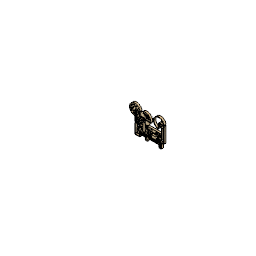
Peças - Texturitas Renders (Autodesk Fusion 360 design; units mm, degrees)
Autodesk Fusion 360 part; units mm, degrees
(part 1 of 2)
sketch "Sketch1" plane through (0, 0, 0) normal (0, 1, 0) x (1, 0, 0) in component "Peça P1"
  line L0 (36, 30) -> (-36, 30)
  line L1 (-40, 26) -> (-40, -6)
  line L2 (40, -6) -> (40, 26)
  arc A0 (-36, 30) -> (-40, 26) centre (-36, 26) ccw
  arc A1 (40, 26) -> (36, 30) centre (36, 26) ccw
  line L3 (-36, -10) -> (-25, -10)
  line L4 (25, -10) -> (36, -10)
  arc A2 (36, -10) -> (40, -6) centre (36, -6) ccw
  arc A3 (-40, -6) -> (-36, -10) centre (-36, -6) ccw
  line L5 (-35, 26) -> (-35, -6)
  line L6 (-38, -6) -> (-38, 26)
  arc A4 (-35, 26) -> (-38, 26) centre (-36.5, 26) ccw
  arc A5 (-38, -6) -> (-35, -6) centre (-36.5, -6) ccw
  line L7 (-30, 26) -> (-30, -6)
  line L8 (-33, -6) -> (-33, 26)
  arc A6 (-30, 26) -> (-33, 26) centre (-31.5, 26) ccw
  arc A7 (-33, -6) -> (-30, -6) centre (-31.5, -6) ccw
  line L9 (-20, 26) -> (-20, 12)
  line L10 (-23, 12) -> (-23, 26)
  arc A8 (-23, 12) -> (-20, 12) centre (-21.5, 12) ccw
  arc A9 (-20, 26) -> (-23, 26) centre (-21.5, 26) ccw
  line L11 (-15, 25) -> (-15, 15)
  line L12 (-18, 15) -> (-18, 25)
  arc A10 (-15, 25) -> (-18, 25) centre (-16.5, 25) ccw
  arc A11 (-18, 15) -> (-15, 15) centre (-16.5, 15) ccw
  line L13 (24.0859, 23.7871) -> (24.0859, 15.7871)
  line L14 (21.0859, 15.7871) -> (21.0859, 23.7871)
  arc A12 (24.0859, 23.7871) -> (21.0859, 23.7871) centre (22.5859, 23.7871) ccw
  arc A13 (21.0859, 15.7871) -> (24.0859, 15.7871) centre (22.5859, 15.7871) ccw
  line L15 (34, 25) -> (34, -5)
  line L16 (31, -5) -> (31, 25)
  arc A14 (34, 25) -> (31, 25) centre (32.5, 25) ccw
  arc A15 (31, -5) -> (34, -5) centre (32.5, -5) ccw
  line L17 (-21, -6) -> (-21, 6)
  arc A16 (-16, 11) -> (-21, 6) centre (-16, 6) ccw
  line L18 (-16, 11) -> (16, 11)
  arc A17 (21, 6) -> (16, 11) centre (16, 6) ccw
  line L19 (21, 6) -> (21, -6)
  arc A18 (-25, -10) -> (-21, -6) centre (-25, -6) ccw
  arc A19 (21, -6) -> (25, -10) centre (25, -6) ccw
  point P0 (-40, 30)
  point P1 (-40, -10)
  point P2 (40, -10)
  point P3 (-20, -10)
  point P4 (-20, 10)
  point P5 (20, 10)
  dimension "d1" = 80
  dimension "d2" = 40
  dimension "d3" = 40
  dimension "d4" = 20
  dimension "d5" = 4
  dimension "d6" = 4
  dimension "d9" = 4
  dimension "d10" = 4
  dimension "d79" = 1.5
  dimension "d80" = 16
  dimension "d81" = 52.5
  dimension "d82" = 47.5
  dimension "d83" = 37.5
  dimension "d84" = 32.5
  dimension "d85" = 16.5
  dimension "d86" = 11
  dimension "d87" = 9.7871
  dimension "d88" = 9
  dimension "d89" = 6.5859
  dimension "d91" = 3
  dimension "d92" = 30
  dimension "d93" = 8
  dimension "d166" = 4
  dimension "d167" = 4
  dimension "d375" = 6
  dimension "d376" = 12
  dimension "d377" = 6
  dimension "d378" = 5
  constraint horizontal L0
  constraint perpendicular L0 L1
  constraint parallel L0 L3
  constraint parallel L1 L2
  constraint coincident P0 L0
  constraint coincident P0 L1
  constraint tangent L0 A0
  constraint tangent L1 A0
  constraint tangent L0 A1
  constraint tangent L2 A1
  constraint collinear L3 L4
  constraint coincident P3 L3
  constraint coincident P2 L2
  constraint coincident P2 L4
  constraint tangent L2 A2
  constraint tangent L4 A2
  constraint coincident P1 L1
  constraint coincident P1 L3
  constraint tangent L1 A3
  constraint tangent L3 A3
  constraint vertical L5
  constraint vertical L6
  constraint tangent L6 A4
  constraint tangent L5 A5
  constraint vertical L7
  constraint vertical L8
  constraint tangent L8 A6
  constraint tangent L7 A7
  constraint vertical L9
  constraint vertical L10
  constraint tangent L10 A8
  constraint tangent L9 A9
  constraint vertical L11
  constraint vertical L12
  constraint tangent L11 A10
  constraint tangent L12 A11
  constraint vertical L13
  constraint vertical L14
  constraint tangent L13 A12
  constraint tangent L13 A13
  constraint vertical L15
  constraint vertical L16
  constraint tangent L15 A14
  constraint tangent L15 A15
  constraint tangent L6 A5
  constraint tangent L5 A4
  constraint tangent L8 A7
  constraint tangent L7 A6
  constraint tangent L10 A9
  constraint tangent L9 A8
  constraint tangent L12 A10
  constraint tangent L11 A11
  constraint tangent L14 A13
  constraint tangent L14 A12
  constraint tangent L16 A15
  constraint tangent L16 A14
  constraint collinear origin P3 P5
  constraint horizontal L1.end L6.start
  constraint horizontal L2.end L5.start
  constraint horizontal L1.end L8.start
  constraint horizontal L2.end L7.start
  constraint horizontal L2.end L9.start
  constraint horizontal L11.start L15.start
  constraint equal A4 A6
  constraint equal A4 A10
  constraint equal A4 A14
  constraint tangent A17 L19
  constraint tangent A16 L18
  constraint tangent L18 A17
  constraint tangent L17 A16
  constraint tangent L17 A18
  constraint tangent L3 A18
  constraint tangent L19 A19
  constraint tangent L4 A19
  constraint parallel L2 L17
  constraint parallel L0 L18
  constraint parallel L1 L19
  constraint equal A4 A8
  constraint equal A16 A17
  constraint equal L3 L4
  constraint equal L1 L18
  constraint vertical P3 L9.end
  constraint vertical P3 P4
  measures "d1" distance of P1 P2
  measures "d2" distance of P0 P1
  measures "d3" distance of P4 P5
  measures "d4" distance of P3 P4
  measures "d5" radius of A0
  measures "d6" radius of A1
  measures "d9" radius of A2
  measures "d10" radius of A3
  measures "d79" radius of A15
  measures "d80" horizontal distance of origin A17.centre
  measures "d81" horizontal distance of A5.centre A17.centre
  measures "d82" horizontal distance of A7.centre A17.centre
  measures "d83" horizontal distance of A8.centre A17.centre
  measures "d84" horizontal distance of A11.centre A17.centre
  measures "d85" horizontal distance of A15.centre A17.centre
  measures "d86" vertical distance of A15.centre A17.centre
  measures "d87" vertical distance of A13.centre A17.centre
  measures "d88" vertical distance of A11.centre A17.centre
  measures "d89" horizontal distance of A13.centre A17.centre
  measures "d91" distance of L13 L14
  measures "d92" vertical distance of A14.centre A15.centre
  measures "d93" vertical distance of A12.centre A13.centre
  measures "d166" radius of A18
  measures "d167" radius of A19
  measures "d375" vertical distance of origin A17.centre
  measures "d376" vertical distance of A5.centre A17.centre
  measures "d377" vertical distance of A8.centre A17.centre
  measures "d378" radius of A17
sketch "Sketch1 (2)" plane through (0, 0, 0) normal (0, 1, 0) x (1, 0, 0) in component "Peça P2"
  arc A0 (36, -10) -> (40, -6) centre (36, -6) ccw
  arc A1 (40, 26) -> (36, 30) centre (36, 26) ccw
  line L0 (40, -6) -> (40, 26)
  line L1 (-40, 26) -> (-40, -6)
  line L2 (-36, -10) -> (-25, -10)
  line L3 (25, -10) -> (36, -10)
  arc A2 (-36, 30) -> (-40, 26) centre (-36, 26) ccw
  arc A3 (-40, -6) -> (-36, -10) centre (-36, -6) ccw
  line L4 (36, 30) -> (-36, 30)
  line L5 (-35, 25) -> (35, 25)
  line L6 (35, 22) -> (-35, 22)
  arc A4 (35, 22) -> (35, 25) centre (35, 23.5) ccw
  arc A5 (-35, 25) -> (-35, 22) centre (-35, 23.5) ccw
  line L7 (-35, 20) -> (35, 20)
  line L8 (35, 17) -> (-35, 17)
  arc A6 (-35, 20) -> (-35, 17) centre (-35, 18.5) ccw
  arc A7 (35, 17) -> (35, 20) centre (35, 18.5) ccw
  line L9 (-34, 14) -> (-34, -5)
  line L10 (-37, -5) -> (-37, 14)
  arc A8 (-34, 14) -> (-37, 14) centre (-35.5, 14) ccw
  arc A9 (-37, -5) -> (-34, -5) centre (-35.5, -5) ccw
  line L11 (34, 10) -> (34, -2)
  line L12 (31, -2) -> (31, 10)
  line L13 (28, 9) -> (28, -1)
  line L14 (25, -1) -> (25, 9)
  arc A10 (28, 9) -> (25, 9) centre (26.5, 9) ccw
  arc A11 (34, 10) -> (31, 10) centre (32.5, 10) ccw
  arc A12 (31, -2) -> (34, -2) centre (32.5, -2) ccw
  arc A13 (25, -1) -> (28, -1) centre (26.5, -1) ccw
  line L15 (-26, 11) -> (-26, 0)
  line L16 (-29, 0) -> (-29, 11)
  arc A14 (-26, 11) -> (-29, 11) centre (-27.5, 11) ccw
  arc A15 (-29, 0) -> (-26, 0) centre (-27.5, 0) ccw
  line L17 (-21, -6) -> (-21, 6)
  arc A16 (-16, 11) -> (-21, 6) centre (-16, 6) ccw
  line L18 (-16, 11) -> (16, 11)
  arc A17 (21, 6) -> (16, 11) centre (16, 6) ccw
  line L19 (21, 6) -> (21, -6)
  arc A18 (21, -6) -> (25, -10) centre (25, -6) ccw
  arc A19 (-25, -10) -> (-21, -6) centre (-25, -6) ccw
  point P0 (-20, -10)
  point P1 (40, -10)
  point P2 (-40, -10)
  point P3 (-40, 30)
  point P4 (20, 10)
  point P5 (-20, 10)
  dimension "d43" = 80
  dimension "d44" = 40
  dimension "d45" = 40
  dimension "d46" = 20
  dimension "d47" = 4
  dimension "d48" = 4
  dimension "d51" = 4
  dimension "d52" = 4
  dimension "d94" = 1.5
  dimension "d95" = 16
  dimension "d96" = 51.5
  dimension "d97" = 43.5
  dimension "d98" = 19
  dimension "d99" = 17.5
  dimension "d100" = 16.5
  dimension "d101" = 12.5
  dimension "d102" = 10.5
  dimension "d103" = 8
  dimension "d104" = 5
  dimension "d105" = 3
  dimension "d106" = 3
  dimension "d107" = 70
  dimension "d108" = 10
  dimension "d169" = 4
  dimension "d170" = 4
  dimension "d393" = 6
  dimension "d394" = 21
  dimension "d395" = 19
  constraint horizontal L4
  constraint perpendicular L1 L4
  constraint parallel L2 L4
  constraint parallel L0 L1
  constraint coincident P3 L4
  constraint coincident P3 L1
  constraint tangent A2 L4
  constraint tangent L1 A2
  constraint tangent A1 L4
  constraint tangent A1 L0
  constraint collinear L2 L3
  constraint coincident P0 L2
  constraint coincident P1 L0
  constraint coincident P1 L3
  constraint tangent A0 L0
  constraint tangent A0 L3
  constraint coincident P2 L1
  constraint coincident P2 L2
  constraint tangent L1 A3
  constraint tangent L2 A3
  constraint horizontal L5
  constraint horizontal L6
  constraint tangent L6 A5
  constraint tangent L6 A4
  constraint horizontal L7
  constraint horizontal L8
  constraint tangent L8 A6
  constraint tangent L8 A7
  constraint vertical L9
  constraint vertical L10
  constraint tangent L10 A8
  constraint tangent L10 A9
  constraint vertical L11
  constraint vertical L12
  constraint vertical L13
  constraint vertical L14
  constraint tangent L13 A10
  constraint tangent L13 A13
  constraint tangent L11 A11
  constraint tangent L11 A12
  constraint vertical L15
  constraint vertical L16
  constraint tangent L16 A14
  constraint tangent L16 A15
  constraint tangent L7 A6
  constraint tangent L5 A5
  constraint tangent L9 A9
  constraint tangent L9 A8
  constraint tangent L15 A15
  constraint tangent L15 A14
  constraint tangent L14 A13
  constraint tangent L14 A10
  constraint tangent L12 A12
  constraint tangent L12 A11
  constraint tangent L7 A7
  constraint tangent L5 A4
  constraint collinear origin P0 P4
  constraint vertical L6.end L8.end
  constraint vertical L5.end L7.end
  constraint equal A4 A9
  constraint equal A4 A12
  constraint equal A4 A13
  constraint equal A4 A15
  constraint horizontal origin L16.start
  constraint tangent L18 A17
  constraint tangent A16 L18
  constraint tangent A17 L19
  constraint tangent L17 A16
  constraint tangent L19 A18
  constraint tangent L3 A18
  constraint tangent L2 A19
  constraint tangent L17 A19
  constraint parallel L0 L17
  constraint parallel L4 L18
  constraint parallel L1 L19
  constraint vertical L14.start A18.centre
  constraint equal L2 L3
  constraint equal L2 L15
  constraint equal L11 L17
  constraint equal L11 L19
  constraint equal L0 L1
  constraint horizontal P5 L11.start
  constraint vertical P0 P5
  constraint horizontal P4 P5
  measures "d43" distance of P1 P2
  measures "d44" distance of P2 P3
  measures "d45" distance of P4 P5
  measures "d46" distance of P0 P5
  measures "d47" radius of A2
  measures "d48" radius of A1
  measures "d51" radius of A0
  measures "d52" radius of A3
  measures "d94" radius of A12
  measures "d95" horizontal distance of origin A17.centre
  measures "d96" horizontal distance of A8.centre A17.centre
  measures "d97" horizontal distance of A14.centre A17.centre
  measures "d98" horizontal distance of A4.centre A17.centre
  measures "d99" vertical distance of A4.centre A17.centre
  measures "d100" horizontal distance of A11.centre A17.centre
  measures "d101" vertical distance of A7.centre A17.centre
  measures "d102" horizontal distance of A10.centre A17.centre
  measures "d103" vertical distance of A8.centre A17.centre
  measures "d104" vertical distance of A14.centre A17.centre
  measures "d105" vertical distance of A10.centre A17.centre
  measures "d106" distance of L7 L8
  measures "d107" horizontal distance of A5.centre A4.centre
  measures "d108" vertical distance of A10.centre A13.centre
  measures "d169" radius of A18
  measures "d170" radius of A19
  measures "d393" vertical distance of origin A17.centre
  measures "d394" distance of L2 A14.centre
  measures "d395" vertical distance of A8.centre A9.centre
sketch "Sketch1 (3)" plane through (0, 0, 0) normal (0, 1, 0) x (1, 0, 0) in component "Peça P3"
  arc A0 (36, -10) -> (40, -6) centre (36, -6) ccw
  arc A1 (40, 26) -> (36, 30) centre (36, 26) ccw
  line L0 (40, -6) -> (40, 26)
  line L1 (-40, 26) -> (-40, -6)
  line L2 (-36, -10) -> (-25, -10)
  line L3 (25, -10) -> (36, -10)
  arc A2 (-36, 30) -> (-40, 26) centre (-36, 26) ccw
  arc A3 (-40, -6) -> (-36, -10) centre (-36, -6) ccw
  line L4 (36, 30) -> (-36, 30)
  circle A4 centre (-32.2316, 20.5441) radius 4.1864
  circle A5 centre (-29.7196, 11.1388) radius 3
  circle A6 centre (-31.076, 0.3956) radius 5
  circle A7 centre (-21.0439, 22.3442) radius 4
  circle A8 centre (-10.8026, 22.2386) radius 3
  circle A9 centre (-14.8673, 15.2035) radius 3
  circle A10 centre (5.8787, 22.2531) radius 3
  circle A11 centre (16.4585, 17.5161) radius 5
  circle A12 centre (30.7592, -0.0073) radius 5
  circle A13 centre (30.6531, 17.2177) radius 3
  circle A14 centre (24.2077, 23.2602) radius 3
  line L5 (-21, -6) -> (-21, 6)
  arc A15 (-16, 11) -> (-21, 6) centre (-16, 6) ccw
  line L6 (-16, 11) -> (16, 11)
  arc A16 (21, 6) -> (16, 11) centre (16, 6) ccw
  line L7 (21, 6) -> (21, -6)
  arc A17 (-25, -10) -> (-21, -6) centre (-25, -6) ccw
  arc A18 (21, -6) -> (25, -10) centre (25, -6) ccw
  point P0 (-20, -10)
  point P1 (40, -10)
  point P2 (-40, -10)
  point P3 (-40, 30)
  point P4 (20, 10)
  point P5 (-20, 10)
  point P6 (-10.8026, 22.2386)
  dimension "d55" = 80
  dimension "d56" = 40
  dimension "d57" = 40
  dimension "d58" = 20
  dimension "d59" = 4
  dimension "d60" = 4
  dimension "d63" = 4
  dimension "d64" = 4
  dimension "d109" = 6
  dimension "d110" = 10
  dimension "d111" = 8
  dimension "d112" = 6
  dimension "d113" = 6
  dimension "d114" = 6
  dimension "d115" = 10
  dimension "d116" = 10
  dimension "d117" = 6
  dimension "d118" = 6
  dimension "d119" = 8.3729
  dimension "d120" = 16
  dimension "d121" = 48.2316
  dimension "d122" = 47.076
  dimension "d123" = 45.7196
  dimension "d124" = 37.0439
  dimension "d125" = 30.8673
  dimension "d126" = 26.8026
  dimension "d127" = 17.2602
  dimension "d128" = 16.3442
  dimension "d129" = 16.2531
  dimension "d130" = 16.2386
  dimension "d131" = 14.7592
  dimension "d132" = 14.6531
  dimension "d133" = 14.5441
  dimension "d134" = 11.5161
  dimension "d135" = 11.2177
  dimension "d136" = 10.1213
  dimension "d137" = 9.2035
  dimension "d138" = 8.2077
  dimension "d139" = 6.0073
  dimension "d140" = 5.6044
  dimension "d141" = 5.1388
  dimension "d142" = 0.4585
  dimension "d172" = 4
  dimension "d173" = 4
  dimension "d390" = 6
  dimension "d391" = 5
  dimension "d392" = 21
  constraint horizontal L4
  constraint perpendicular L1 L4
  constraint parallel L2 L4
  constraint parallel L0 L1
  constraint coincident P3 L4
  constraint coincident P3 L1
  constraint tangent A2 L4
  constraint tangent L1 A2
  constraint tangent A1 L4
  constraint tangent A1 L0
  constraint collinear L2 L3
  constraint coincident P0 L2
  constraint coincident P1 L0
  constraint coincident P1 L3
  constraint tangent A0 L0
  constraint tangent A0 L3
  constraint coincident P2 L1
  constraint coincident P2 L2
  constraint tangent L1 A3
  constraint tangent L2 A3
  constraint coincident P6 A8.centre
  constraint collinear origin P0 P4
  constraint tangent A16 L7
  constraint tangent A15 L6
  constraint tangent L6 A16
  constraint tangent L5 A15
  constraint tangent L2 A17
  constraint tangent L5 A17
  constraint tangent L7 A18
  constraint tangent L3 A18
  constraint parallel L0 L5
  constraint parallel L4 L6
  constraint parallel L1 L7
  constraint equal A15 A16
  constraint equal L2 L3
  constraint equal L0 L6
  constraint horizontal A0.start P2
  constraint vertical P0 P5
  constraint horizontal P4 P5
  measures "d55" distance of P1 P2
  measures "d56" distance of P2 P3
  measures "d57" distance of P4 P5
  measures "d58" distance of P0 P5
  measures "d59" radius of A2
  measures "d60" radius of A1
  measures "d63" radius of A0
  measures "d64" radius of A3
  measures "d109" diameter of A5
  measures "d110" diameter of A6
  measures "d111" diameter of A7
  measures "d112" diameter of A8
  measures "d113" diameter of A9
  measures "d114" diameter of A10
  measures "d115" diameter of A11
  measures "d116" diameter of A12
  measures "d117" diameter of A13
  measures "d118" diameter of A14
  measures "d119" diameter of A4
  measures "d120" horizontal distance of origin A16.centre
  measures "d121" horizontal distance of A4.centre A16.centre
  measures "d122" horizontal distance of A6.centre A16.centre
  measures "d123" horizontal distance of A5.centre A16.centre
  measures "d124" horizontal distance of A7.centre A16.centre
  measures "d125" horizontal distance of A9.centre A16.centre
  measures "d126" horizontal distance of P6 A16.centre
  measures "d127" vertical distance of A14.centre A16.centre
  measures "d128" vertical distance of A7.centre A16.centre
  measures "d129" vertical distance of A10.centre A16.centre
  measures "d130" vertical distance of P6 A16.centre
  measures "d131" horizontal distance of A12.centre A16.centre
  measures "d132" horizontal distance of A13.centre A16.centre
  measures "d133" vertical distance of A4.centre A16.centre
  measures "d134" vertical distance of A11.centre A16.centre
  measures "d135" vertical distance of A13.centre A16.centre
  measures "d136" horizontal distance of A10.centre A16.centre
  measures "d137" vertical distance of A9.centre A16.centre
  measures "d138" horizontal distance of A14.centre A16.centre
  measures "d139" vertical distance of A12.centre A16.centre
  measures "d140" vertical distance of A6.centre A16.centre
  measures "d141" vertical distance of A5.centre A16.centre
  measures "d142" horizontal distance of A11.centre A16.centre
  measures "d172" radius of A17
  measures "d173" radius of A18
  measures "d390" vertical distance of origin A16.centre
  measures "d391" radius of A16
  measures "d392" distance of P1 L6
sketch "Sketch1 (4)" plane through (0, 0, 0) normal (0, 1, 0) x (1, 0, 0) in component "Peça P4"
  arc A0 (36, -10) -> (40, -6) centre (36, -6) ccw
  arc A1 (40, 26) -> (36, 30) centre (36, 26) ccw
  line L0 (40, -6) -> (40, 26)
  line L1 (-40, 26) -> (-40, -6)
  line L2 (-36, -10) -> (-25, -10)
  line L3 (25, -10) -> (36, -10)
  arc A2 (-36, 30) -> (-40, 26) centre (-36, 26) ccw
  arc A3 (-40, -6) -> (-36, -10) centre (-36, -6) ccw
  line L4 (36, 30) -> (-36, 30)
  line L5 (-24, -2) -> (-24, 6)
  arc A4 (-16, 14) -> (-24, 6) centre (-16, 6) ccw
  line L6 (-16, 14) -> (16, 14)
  arc A5 (24, 6) -> (16, 14) centre (16, 6) ccw
  line L7 (24, 6) -> (24, -2)
  line L8 (28, -6) -> (32, -6)
  line L9 (36, -2) -> (36, 22)
  line L10 (32, 26) -> (-32, 26)
  line L11 (-36, 22) -> (-36, -2)
  line L12 (-32, -6) -> (-28, -6)
  arc A6 (36, 22) -> (32, 26) centre (32, 22) ccw
  arc A7 (-32, 26) -> (-36, 22) centre (-32, 22) ccw
  arc A8 (-36, -2) -> (-32, -6) centre (-32, -2) ccw
  arc A9 (-28, -6) -> (-24, -2) centre (-28, -2) ccw
  arc A10 (24, -2) -> (28, -6) centre (28, -2) ccw
  arc A11 (32, -6) -> (36, -2) centre (32, -2) ccw
  line L13 (-21, -6) -> (-21, 6)
  arc A12 (-16, 11) -> (-21, 6) centre (-16, 6) ccw
  line L14 (-16, 11) -> (16, 11)
  arc A13 (21, 6) -> (16, 11) centre (16, 6) ccw
  line L15 (21, 6) -> (21, -6)
  arc A14 (-25, -10) -> (-21, -6) centre (-25, -6) ccw
  arc A15 (21, -6) -> (25, -10) centre (25, -6) ccw
  point P0 (-20, -10)
  point P1 (40, -10)
  point P2 (-40, -10)
  point P3 (-40, 30)
  point P4 (20, 10)
  dimension "d67" = 80
  dimension "d68" = 40
  dimension "d71" = 4
  dimension "d72" = 4
  dimension "d75" = 4
  dimension "d76" = 4
  dimension "d144" = 16
  dimension "d149" = 4
  dimension "d150" = 4
  dimension "d151" = 4
  dimension "d152" = 4
  dimension "d153" = 4
  dimension "d154" = 4
  dimension "d155" = 6
  dimension "d175" = 4
  dimension "d176" = 4
  dimension "d379" = 40
  dimension "d380" = 10
  dimension "d381" = 20
  dimension "d382" = 3
  dimension "d383" = 3
  dimension "d384" = 3
  dimension "d385" = 5
  dimension "d386" = 16
  dimension "d387" = 8
  dimension "d388" = 16
  dimension "d389" = 4
  constraint horizontal L4
  constraint perpendicular L1 L4
  constraint parallel L2 L4
  constraint parallel L0 L1
  constraint coincident P3 L4
  constraint coincident P3 L1
  constraint tangent A2 L4
  constraint tangent L1 A2
  constraint tangent A1 L4
  constraint tangent A1 L0
  constraint collinear L2 L3
  constraint coincident P0 L2
  constraint coincident P1 L0
  constraint coincident P1 L3
  constraint tangent A0 L0
  constraint tangent A0 L3
  constraint coincident P2 L1
  constraint coincident P2 L2
  constraint tangent L1 A3
  constraint tangent L2 A3
  constraint collinear origin P0 P4
  constraint tangent A5 L7
  constraint tangent L6 A5
  constraint tangent A4 L6
  constraint tangent L5 A4
  constraint tangent L9 A6
  constraint tangent L10 A6
  constraint tangent L10 A7
  constraint tangent L11 A7
  constraint tangent L11 A8
  constraint tangent L12 A8
  constraint tangent L5 A9
  constraint tangent L12 A9
  constraint tangent L7 A10
  constraint tangent L8 A10
  constraint tangent L8 A11
  constraint tangent L9 A11
  constraint parallel L0 L5
  constraint tangent L2 A14
  constraint tangent L13 A14
  constraint tangent L15 A15
  constraint tangent L3 A15
  constraint tangent L13 A12
  constraint tangent L14 A13
  constraint tangent A12 L14
  constraint tangent A13 L15
  constraint parallel L4 L6
  constraint equal A12 A13
  measures "d67" distance of P1 P2
  measures "d68" distance of P2 P3
  measures "d71" radius of A2
  measures "d72" radius of A1
  measures "d75" radius of A0
  measures "d76" radius of A3
  measures "d144" horizontal distance of origin A5.centre
  measures "d149" radius of A6
  measures "d150" radius of A7
  measures "d151" radius of A8
  measures "d152" radius of A9
  measures "d153" radius of A10
  measures "d154" radius of A11
  measures "d155" vertical distance of origin A5.centre
  measures "d175" radius of A14
  measures "d176" radius of A15
  measures "d379" distance of origin L1
  measures "d380" distance of origin L2
  measures "d381" horizontal distance of P0 P2
  measures "d382" distance of L5 L13
  measures "d383" distance of L6 L14
  measures "d384" distance of L7 L15
  measures "d385" radius of A13
  measures "d386" distance of L0 L7
  measures "d387" radius of A4
  measures "d388" horizontal distance of origin A4.centre
  measures "d389" horizontal distance of P4 A5.centre
sketch "Sketch G2" plane through (0, 0, 0) normal (0, 1, 0) x (1, 0, 0) in component "Peça G2"
  line L0 (9.5, 4) -> (9.5, 36)
  line L1 (5.5, 40) -> (-106.5, 40)
  line L2 (-110.5, 36) -> (-110.5, 4)
  line L3 (-87.5, 21) -> (-13.5, 21)
  line L4 (-9.5, 17) -> (-9.5, 4)
  line L5 (-91.5, 4) -> (-91.5, 17)
  line L6 (-106.5, 0) -> (-95.5, 0)
  line L7 (-5.5, 0) -> (5.5, 0)
  arc A0 (-95.5, 0) -> (-91.5, 4) centre (-95.5, 4) ccw
  arc A1 (-110.5, 4) -> (-106.5, 0) centre (-106.5, 4) ccw
  arc A2 (-106.5, 40) -> (-110.5, 36) centre (-106.5, 36) ccw
  arc A3 (-87.5, 21) -> (-91.5, 17) centre (-87.5, 17) ccw
  arc A4 (-9.5, 17) -> (-13.5, 21) centre (-13.5, 17) ccw
  arc A5 (9.5, 36) -> (5.5, 40) centre (5.5, 36) ccw
  arc A6 (5.5, 0) -> (9.5, 4) centre (5.5, 4) ccw
  arc A7 (-9.5, 4) -> (-5.5, 0) centre (-5.5, 4) ccw
  line L8 (-103, 35) -> (-103, 4)
  line L9 (-106, 4) -> (-106, 35)
  line L10 (-98, 35) -> (-98, 22)
  line L11 (-101, 22) -> (-101, 35)
  line L12 (-5, 35) -> (-5, 25)
  line L13 (-8, 25) -> (-8, 35)
  line L14 (0, 35) -> (0, 5)
  line L15 (-3, 5) -> (-3, 35)
  arc A8 (-5, 35) -> (-8, 35) centre (-6.5, 35) ccw
  arc A9 (-8, 25) -> (-5, 25) centre (-6.5, 25) ccw
  arc A10 (0, 35) -> (-3, 35) centre (-1.5, 35) ccw
  arc A11 (-3, 5) -> (0, 5) centre (-1.5, 5) ccw
  arc A12 (-106, 4) -> (-103, 4) centre (-104.5, 4) ccw
  arc A13 (-103, 35) -> (-106, 35) centre (-104.5, 35) ccw
  arc A14 (-98, 35) -> (-101, 35) centre (-99.5, 35) ccw
  arc A15 (-101, 22) -> (-98, 22) centre (-99.5, 22) ccw
  line L16 (-92, 35) -> (-13, 35)
  line L17 (-13, 32) -> (-92, 32)
  line L18 (-85, 30) -> (-18, 30)
  line L19 (-18, 27) -> (-85, 27)
  arc A16 (-92, 35) -> (-92, 32) centre (-92, 33.5) ccw
  arc A17 (-13, 32) -> (-13, 35) centre (-13, 33.5) ccw
  arc A18 (-18, 27) -> (-18, 30) centre (-18, 28.5) ccw
  arc A19 (-85, 30) -> (-85, 27) centre (-85, 28.5) ccw
  line L20 (5, 35) -> (5, 5)
  line L21 (2, 5) -> (2, 35)
  arc A20 (5, 35) -> (2, 35) centre (3.5, 35) ccw
  arc A21 (2, 5) -> (5, 5) centre (3.5, 5) ccw
  point P0 (9.5, 0)
  point P1 (9.5, 40)
  point P2 (-110.5, 40)
  point P3 (-91.5, 21)
  point P4 (-9.5, 21)
  point P5 (-91.5, 0)
  dimension "d177" = 120
  dimension "d178" = 40
  dimension "d179" = 82
  dimension "d180" = 21
  dimension "d181" = 4
  dimension "d182" = 4
  dimension "d183" = 4
  dimension "d184" = 4
  dimension "d185" = 4
  dimension "d186" = 4
  dimension "d187" = 4
  dimension "d188" = 4
  dimension "d240" = 1.5
  dimension "d241" = 1.5
  dimension "d242" = 5
  dimension "d243" = 4
  dimension "d244" = 1
  dimension "d245" = 103
  dimension "d246" = 98
  dimension "d247" = 28.5
  dimension "d248" = 23.5
  dimension "d249" = 20
  dimension "d250" = 17
  dimension "d251" = 16.5
  dimension "d252" = 11.5
  dimension "d253" = 5
  dimension "d254" = 3
  dimension "d255" = 3
  dimension "d256" = 3
  dimension "d257" = 79
  dimension "d258" = 67
  constraint horizontal L6
  constraint perpendicular L0 L7
  constraint parallel L1 L6
  constraint parallel L0 L2
  constraint horizontal L3
  constraint vertical L4
  constraint vertical L5
  constraint collinear L6 L7
  constraint coincident P5 L5
  constraint coincident P5 L6
  constraint tangent L5 A0
  constraint tangent L6 A0
  constraint tangent L2 A1
  constraint tangent L6 A1
  constraint coincident P2 L1
  constraint coincident P2 L2
  constraint tangent L1 A2
  constraint tangent L2 A2
  constraint coincident P3 L3
  constraint coincident P3 L5
  constraint tangent L3 A3
  constraint tangent L5 A3
  constraint coincident P4 L3
  constraint coincident P4 L4
  constraint tangent L3 A4
  constraint tangent L4 A4
  constraint coincident P1 L0
  constraint coincident P1 L1
  constraint tangent L0 A5
  constraint tangent L1 A5
  constraint coincident origin L7
  constraint coincident P0 L0
  constraint coincident P0 L7
  constraint tangent L0 A6
  constraint tangent L7 A6
  constraint tangent L4 A7
  constraint tangent L7 A7
  constraint vertical L8
  constraint vertical L9
  constraint vertical L10
  constraint vertical L11
  constraint tangent L9 A13
  constraint tangent L9 A12
  constraint tangent L10 A14
  constraint tangent L11 A15
  constraint vertical L12
  constraint vertical L13
  constraint vertical L14
  constraint vertical L15
  constraint tangent L13 A8
  constraint tangent L13 A9
  constraint tangent L14 A10
  constraint tangent L15 A11
  constraint horizontal L16
  constraint horizontal L17
  constraint horizontal L18
  constraint horizontal L19
  constraint tangent L17 A16
  constraint tangent L19 A19
  constraint tangent L19 A18
  constraint tangent L17 A17
  constraint vertical L20
  constraint vertical L21
  constraint tangent L20 A20
  constraint tangent L21 A21
  constraint tangent L8 A12
  constraint tangent L8 A13
  constraint tangent L11 A14
  constraint tangent L10 A15
  constraint tangent L16 A16
  constraint tangent L18 A19
  constraint tangent L18 A18
  constraint tangent L16 A17
  constraint tangent L12 A9
  constraint tangent L12 A8
  constraint tangent L15 A10
  constraint tangent L14 A11
  constraint tangent L21 A20
  constraint tangent L20 A21
  constraint horizontal L2.end L9.start
  constraint horizontal L8.start L10.start
  constraint horizontal L8.start L16.start
  constraint horizontal L8.start L12.start
  constraint horizontal L8.start L14.start
  constraint horizontal L8.start L20.start
  constraint horizontal L15.start L21.start
  constraint equal A8 A12
  constraint equal A8 A14
  constraint equal A8 A20
  constraint equal L6 L7
  measures "d177" distance of P1 P2
  measures "d178" distance of P0 P1
  measures "d179" distance of P3 P4
  measures "d180" distance of P3 P5
  measures "d181" radius of A0
  measures "d182" radius of A1
  measures "d183" radius of A2
  measures "d184" radius of A3
  measures "d185" radius of A4
  measures "d186" radius of A5
  measures "d187" radius of A6
  measures "d188" radius of A7
  measures "d240" radius of A21
  measures "d241" horizontal distance of origin A11.centre
  measures "d242" horizontal distance of A11.centre A21.centre
  measures "d243" horizontal distance of A7.centre A11.centre
  measures "d244" vertical distance of A7.centre A11.centre
  measures "d245" horizontal distance of A12.centre A11.centre
  measures "d246" horizontal distance of A15.centre A11.centre
  measures "d247" vertical distance of A11.centre A17.centre
  measures "d248" vertical distance of A11.centre A18.centre
  measures "d249" vertical distance of A9.centre A11.centre
  measures "d250" vertical distance of A15.centre A11.centre
  measures "d251" horizontal distance of A11.centre A18.centre
  measures "d252" horizontal distance of A11.centre A17.centre
  measures "d253" horizontal distance of A9.centre A11.centre
  measures "d254" distance of L16 L17
  measures "d255" distance of L18 L19
  measures "d256" distance of L14 L15
  measures "d257" horizontal distance of A16.centre A17.centre
  measures "d258" horizontal distance of A19.centre A18.centre
sketch "Sketch1 (5)" plane through (0, 0, 0) normal (0, 1, 0) x (1, 0, 0) in component "Peça G1"
  arc A0 (-9.5, 4) -> (-5.5, 0) centre (-5.5, 4) ccw
  arc A1 (-106.5, 40) -> (-110.5, 36) centre (-106.5, 36) ccw
  line L0 (-87.5, 21) -> (-13.5, 21)
  arc A2 (-9.5, 17) -> (-13.5, 21) centre (-13.5, 17) ccw
  arc A3 (-95.5, 0) -> (-91.5, 4) centre (-95.5, 4) ccw
  arc A4 (-110.5, 4) -> (-106.5, 0) centre (-106.5, 4) ccw
  arc A5 (9.5, 36) -> (5.5, 40) centre (5.5, 36) ccw
  line L1 (-5.5, 0) -> (5.5, 0)
  line L2 (-110.5, 36) -> (-110.5, 4)
  line L3 (-9.5, 17) -> (-9.5, 4)
  line L4 (-106.5, 0) -> (-95.5, 0)
  arc A6 (-87.5, 21) -> (-91.5, 17) centre (-87.5, 17) ccw
  line L5 (5.5, 40) -> (-106.5, 40)
  line L6 (-91.5, 4) -> (-91.5, 17)
  line L7 (9.5, 4) -> (9.5, 36)
  arc A7 (5.5, 0) -> (9.5, 4) centre (5.5, 4) ccw
  arc A8 (-106, 35) -> (-109, 35) centre (-107.5, 35) ccw
  line L8 (-101, 35) -> (-101, 5)
  line L9 (-104, 5) -> (-104, 35)
  arc A9 (-101, 35) -> (-104, 35) centre (-102.5, 35) ccw
  arc A10 (-104, 5) -> (-101, 5) centre (-102.5, 5) ccw
  line L10 (-109, 35) -> (-109, 12)
  line L11 (-106, 12) -> (-106, 35)
  arc A11 (-109, 12) -> (-106, 12) centre (-107.5, 12) ccw
  line L12 (-95, 35) -> (-95, 24)
  line L13 (-98, 24) -> (-98, 35)
  arc A12 (-95, 35) -> (-98, 35) centre (-96.5, 35) ccw
  arc A13 (-98, 24) -> (-95, 24) centre (-96.5, 24) ccw
  line L14 (-85, 35) -> (-85, 27)
  line L15 (-88, 27) -> (-88, 35)
  arc A14 (-85, 35) -> (-88, 35) centre (-86.5, 35) ccw
  arc A15 (-88, 27) -> (-85, 27) centre (-86.5, 27) ccw
  line L16 (-80, 35) -> (-80, 27)
  line L17 (-83, 27) -> (-83, 35)
  arc A16 (-80, 35) -> (-83, 35) centre (-81.5, 35) ccw
  arc A17 (-83, 27) -> (-80, 27) centre (-81.5, 27) ccw
  line L18 (-15, 35) -> (-15, 27)
  line L19 (-18, 27) -> (-18, 35)
  arc A18 (-15, 35) -> (-18, 35) centre (-16.5, 35) ccw
  arc A19 (-18, 27) -> (-15, 27) centre (-16.5, 27) ccw
  line L20 (-10, 35) -> (-10, 27)
  line L21 (-13, 27) -> (-13, 35)
  line L22 (-3, 35) -> (-3, 5)
  line L23 (-6, 5) -> (-6, 35)
  line L24 (3, 35) -> (3, 5)
  line L25 (0, 5) -> (0, 35)
  arc A20 (-10, 35) -> (-13, 35) centre (-11.5, 35) ccw
  arc A21 (-13, 27) -> (-10, 27) centre (-11.5, 27) ccw
  arc A22 (3, 35) -> (0, 35) centre (1.5, 35) ccw
  arc A23 (-3, 35) -> (-6, 35) centre (-4.5, 35) ccw
  arc A24 (-6, 5) -> (-3, 5) centre (-4.5, 5) ccw
  arc A25 (0, 5) -> (3, 5) centre (1.5, 5) ccw
  point P0 (-110.5, 40)
  point P1 (-9.5, 21)
  point P2 (-91.5, 21)
  point P3 (-91.5, 0)
  point P4 (9.5, 0)
  point P5 (9.5, 40)
  dimension "d189" = 120
  dimension "d190" = 40
  dimension "d191" = 82
  dimension "d192" = 21
  dimension "d193" = 4
  dimension "d194" = 4
  dimension "d195" = 4
  dimension "d196" = 4
  dimension "d197" = 4
  dimension "d198" = 4
  dimension "d199" = 4
  dimension "d200" = 4
  dimension "d225" = 1.5
  dimension "d226" = 1.5
  dimension "d227" = 104
  dimension "d228" = 6
  dimension "d229" = 4
  dimension "d230" = 1
  dimension "d231" = 109
  dimension "d232" = 98
  dimension "d233" = 88
  dimension "d234" = 83
  dimension "d235" = 22
  dimension "d236" = 19
  dimension "d237" = 18
  dimension "d238" = 13
  dimension "d239" = 7
  constraint horizontal L4
  constraint perpendicular L1 L7
  constraint parallel L4 L5
  constraint parallel L2 L7
  constraint horizontal L0
  constraint vertical L3
  constraint vertical L6
  constraint collinear L1 L4
  constraint coincident P3 L6
  constraint coincident P3 L4
  constraint tangent A3 L6
  constraint tangent A3 L4
  constraint tangent A4 L2
  constraint tangent A4 L4
  constraint coincident P0 L5
  constraint coincident P0 L2
  constraint tangent A1 L5
  constraint tangent A1 L2
  constraint coincident P2 L0
  constraint coincident P2 L6
  constraint tangent L0 A6
  constraint tangent A6 L6
  constraint coincident P1 L0
  constraint coincident P1 L3
  constraint tangent L0 A2
  constraint tangent A2 L3
  constraint coincident P5 L7
  constraint coincident P5 L5
  constraint tangent A5 L7
  constraint tangent A5 L5
  constraint coincident origin L1
  constraint coincident P4 L7
  constraint coincident P4 L1
  constraint tangent L7 A7
  constraint tangent L1 A7
  constraint tangent A0 L3
  constraint tangent A0 L1
  constraint vertical L8
  constraint vertical L9
  constraint tangent L8 A9
  constraint tangent L9 A10
  constraint tangent A8 L10
  constraint vertical L10
  constraint tangent A8 L11
  constraint tangent L11 A11
  constraint vertical L12
  constraint vertical L13
  constraint tangent L12 A12
  constraint tangent L13 A13
  constraint vertical L14
  constraint vertical L15
  constraint tangent L15 A14
  constraint tangent L14 A15
  constraint vertical L16
  constraint vertical L17
  constraint tangent L16 A16
  constraint tangent L16 A17
  constraint vertical L18
  constraint vertical L19
  constraint tangent L18 A18
  constraint tangent L18 A19
  constraint vertical L20
  constraint vertical L21
  constraint vertical L22
  constraint vertical L23
  constraint vertical L24
  constraint vertical L25
  constraint tangent L22 A23
  constraint tangent L22 A24
  constraint tangent L24 A22
  constraint tangent L24 A25
  constraint tangent L20 A20
  constraint tangent L21 A21
  constraint tangent L10 A11
  constraint tangent L9 A9
  constraint tangent L8 A10
  constraint tangent L13 A12
  constraint tangent L12 A13
  constraint tangent L15 A15
  constraint tangent L14 A14
  constraint tangent L17 A17
  constraint tangent L17 A16
  constraint tangent L19 A19
  constraint tangent L19 A18
  constraint tangent L21 A20
  constraint tangent L20 A21
  constraint tangent L23 A24
  constraint tangent L23 A23
  constraint tangent L25 A25
  constraint tangent L25 A22
  constraint parallel L10 L11
  constraint horizontal A8.start L8.start
  constraint horizontal A8.start L12.start
  constraint horizontal A8.start L14.start
  constraint horizontal A8.start L16.start
  constraint horizontal A8.start L18.start
  constraint horizontal A8.start L20.start
  constraint horizontal A8.start L22.start
  constraint horizontal A8.start L24.start
  constraint horizontal L9.start L23.start
  constraint horizontal L9.start L25.start
  constraint horizontal L15.start L17.start
  constraint horizontal L15.start L19.start
  constraint horizontal L15.start L21.start
  constraint equal A8 A9
  constraint equal A8 A12
  constraint equal A8 A14
  constraint equal A8 A16
  constraint equal A8 A18
  constraint equal A8 A20
  constraint equal A8 A22
  constraint equal A8 A23
  constraint equal L1 L4
  constraint equal L1 L12
  measures "d189" distance of P0 P5
  measures "d190" distance of P4 P5
  measures "d191" distance of P1 P2
  measures "d192" distance of P2 P3
  measures "d193" radius of A3
  measures "d194" radius of A4
  measures "d195" radius of A1
  measures "d196" radius of A6
  measures "d197" radius of A2
  measures "d198" radius of A5
  measures "d199" radius of A7
  measures "d200" radius of A0
  measures "d225" radius of A25
  measures "d226" horizontal distance of origin A25.centre
  measures "d227" horizontal distance of A10.centre A25.centre
  measures "d228" horizontal distance of A24.centre A25.centre
  measures "d229" horizontal distance of A7.centre A25.centre
  measures "d230" vertical distance of A7.centre A25.centre
  measures "d231" horizontal distance of A11.centre A25.centre
  measures "d232" horizontal distance of A13.centre A25.centre
  measures "d233" horizontal distance of A15.centre A25.centre
  measures "d234" horizontal distance of A17.centre A25.centre
  measures "d235" vertical distance of A25.centre A21.centre
  measures "d236" vertical distance of A13.centre A25.centre
  measures "d237" horizontal distance of A19.centre A25.centre
  measures "d238" horizontal distance of A25.centre A21.centre
  measures "d239" vertical distance of A11.centre A25.centre
sketch "Sketch G3" plane through (0, 0, 0) normal (0, 1, 0) x (1, 0, 0) in component "Peça G3"
  line L0 (-91.5, 4) -> (-91.5, 17)
  arc A0 (9.5, 36) -> (5.5, 40) centre (5.5, 36) ccw
  arc A1 (-95.5, 0) -> (-91.5, 4) centre (-95.5, 4) ccw
  line L1 (-106.5, 0) -> (-95.5, 0)
  line L2 (9.5, 4) -> (9.5, 36)
  line L3 (-87.5, 21) -> (-13.5, 21)
  arc A2 (-87.5, 21) -> (-91.5, 17) centre (-87.5, 17) ccw
  line L4 (-5.5, 0) -> (5.5, 0)
  arc A3 (-110.5, 4) -> (-106.5, 0) centre (-106.5, 4) ccw
  line L5 (5.5, 40) -> (-106.5, 40)
  arc A4 (-9.5, 17) -> (-13.5, 21) centre (-13.5, 17) ccw
  arc A5 (-106.5, 40) -> (-110.5, 36) centre (-106.5, 36) ccw
  line L6 (-9.5, 17) -> (-9.5, 4)
  arc A6 (5.5, 0) -> (9.5, 4) centre (5.5, 4) ccw
  arc A7 (-9.5, 4) -> (-5.5, 0) centre (-5.5, 4) ccw
  line L7 (-110.5, 36) -> (-110.5, 4)
  circle A8 centre (-102.8112, 31.3685) radius 5
  circle A9 centre (-92.954, 32.705) radius 3
  circle A10 centre (-104.4819, 22.3467) radius 3
  circle A11 centre (-68.9269, 26.9274) radius 3
  circle A12 centre (-82.9299, 29.5307) radius 4
  circle A13 centre (-37.621, 31.6914) radius 4
  circle A14 centre (-21.7411, 28.5154) radius 3
  circle A15 centre (-73.741, 32.8721) radius 3
  circle A16 centre (-7.9155, 31.8697) radius 5
  circle A17 centre (3.4398, 26.2469) radius 4
  circle A18 centre (-5.3185, 22.2959) radius 3
  circle A19 centre (1.625, 34.4137) radius 3
  circle A20 centre (-0.7814, 16.8514) radius 3
  circle A21 centre (-95.8614, 23.7078) radius 3
  circle A22 centre (-100.8514, 14.5583) radius 4
  point P0 (-110.5, 40)
  point P1 (-9.5, 21)
  point P2 (-91.5, 21)
  point P3 (-91.5, 0)
  point P4 (9.5, 0)
  point P5 (9.5, 40)
  dimension "d259" = 120
  dimension "d260" = 40
  dimension "d261" = 82
  dimension "d262" = 21
  dimension "d263" = 4
  dimension "d264" = 4
  dimension "d265" = 4
  dimension "d266" = 4
  dimension "d267" = 4
  dimension "d268" = 4
  dimension "d269" = 4
  dimension "d270" = 4
  dimension "d290" = 10
  dimension "d291" = 6
  dimension "d292" = 6
  dimension "d293" = 6
  dimension "d294" = 8
  dimension "d295" = 8
  dimension "d296" = 6
  dimension "d297" = 6
  dimension "d298" = 10
  dimension "d299" = 8
  dimension "d300" = 6
  dimension "d301" = 6
  dimension "d302" = 6
  dimension "d303" = 6
  dimension "d304" = 8
  dimension "d305" = 5.5
  dimension "d306" = 109.9819
  dimension "d307" = 108.3112
  dimension "d308" = 106.3514
  dimension "d309" = 101.3614
  dimension "d310" = 98.454
  dimension "d311" = 88.4299
  dimension "d312" = 79.241
  dimension "d313" = 74.4269
  dimension "d314" = 43.121
  dimension "d315" = 30.4137
  dimension "d316" = 28.8721
  dimension "d317" = 28.705
  dimension "d318" = 27.8697
  dimension "d319" = 27.6914
  dimension "d320" = 27.3685
  dimension "d321" = 27.2411
  dimension "d322" = 25.5307
  dimension "d323" = 24.5154
  dimension "d324" = 22.9274
  dimension "d325" = 22.2469
  dimension "d326" = 19.7078
  dimension "d327" = 18.3467
  dimension "d328" = 18.2959
  dimension "d329" = 13.4155
  dimension "d330" = 12.8514
  dimension "d331" = 10.8185
  dimension "d332" = 10.5583
  dimension "d333" = 6.2814
  dimension "d334" = 3.875
  dimension "d335" = 2.0602
  constraint horizontal L1
  constraint perpendicular L2 L4
  constraint parallel L1 L5
  constraint parallel L2 L7
  constraint horizontal L3
  constraint vertical L6
  constraint vertical L0
  constraint collinear L1 L4
  constraint coincident P3 L0
  constraint coincident P3 L1
  constraint tangent L0 A1
  constraint tangent A1 L1
  constraint tangent A3 L7
  constraint tangent L1 A3
  constraint coincident P0 L5
  constraint coincident P0 L7
  constraint tangent L5 A5
  constraint tangent A5 L7
  constraint coincident P2 L3
  constraint coincident P2 L0
  constraint tangent L3 A2
  constraint tangent L0 A2
  constraint coincident P1 L3
  constraint coincident P1 L6
  constraint tangent L3 A4
  constraint tangent A4 L6
  constraint coincident P5 L2
  constraint coincident P5 L5
  constraint tangent A0 L2
  constraint tangent A0 L5
  constraint coincident origin L4
  constraint coincident P4 L2
  constraint coincident P4 L4
  constraint tangent L2 A6
  constraint tangent L4 A6
  constraint tangent L6 A7
  constraint tangent L4 A7
  constraint equal L1 L4
  measures "d259" distance of P0 P5
  measures "d260" distance of P4 P5
  measures "d261" distance of P1 P2
  measures "d262" distance of P2 P3
  measures "d263" radius of A1
  measures "d264" radius of A3
  measures "d265" radius of A5
  measures "d266" radius of A2
  measures "d267" radius of A4
  measures "d268" radius of A0
  measures "d269" radius of A6
  measures "d270" radius of A7
  measures "d290" diameter of A8
  measures "d291" diameter of A9
  measures "d292" diameter of A10
  measures "d293" diameter of A11
  measures "d294" diameter of A12
  measures "d295" diameter of A13
  measures "d296" diameter of A14
  measures "d297" diameter of A15
  measures "d298" diameter of A16
  measures "d299" diameter of A17
  measures "d300" diameter of A18
  measures "d301" diameter of A19
  measures "d302" diameter of A20
  measures "d303" diameter of A21
  measures "d304" diameter of A22
  measures "d305" horizontal distance of origin A6.centre
  measures "d306" horizontal distance of A6.centre A10.centre
  measures "d307" horizontal distance of A6.centre A8.centre
  measures "d308" horizontal distance of A6.centre A22.centre
  measures "d309" horizontal distance of A6.centre A21.centre
  measures "d310" horizontal distance of A6.centre A9.centre
  measures "d311" horizontal distance of A6.centre A12.centre
  measures "d312" horizontal distance of A6.centre A15.centre
  measures "d313" horizontal distance of A6.centre A11.centre
  measures "d314" horizontal distance of A6.centre A13.centre
  measures "d315" vertical distance of A6.centre A19.centre
  measures "d316" vertical distance of A6.centre A15.centre
  measures "d317" vertical distance of A6.centre A9.centre
  measures "d318" vertical distance of A6.centre A16.centre
  measures "d319" vertical distance of A6.centre A13.centre
  measures "d320" vertical distance of A6.centre A8.centre
  measures "d321" horizontal distance of A6.centre A14.centre
  measures "d322" vertical distance of A6.centre A12.centre
  measures "d323" vertical distance of A6.centre A14.centre
  measures "d324" vertical distance of A6.centre A11.centre
  measures "d325" vertical distance of A6.centre A17.centre
  measures "d326" vertical distance of A6.centre A21.centre
  measures "d327" vertical distance of A6.centre A10.centre
  measures "d328" vertical distance of A6.centre A18.centre
  measures "d329" horizontal distance of A6.centre A16.centre
  measures "d330" vertical distance of A6.centre A20.centre
  measures "d331" horizontal distance of A6.centre A18.centre
  measures "d332" vertical distance of A6.centre A22.centre
  measures "d333" horizontal distance of A6.centre A20.centre
  measures "d334" horizontal distance of A6.centre A19.centre
  measures "d335" horizontal distance of A6.centre A17.centre
sketch "Sketch G4" plane through (0, 0, 0) normal (0, 1, 0) x (1, 0, 0) in component "Peça G4"
  arc A0 (9.5, 36) -> (5.5, 40) centre (5.5, 36) ccw
  line L0 (-87.5, 21) -> (-13.5, 21)
  line L1 (-9.5, 17) -> (-9.5, 4)
  line L2 (-106.5, 0) -> (-95.5, 0)
  arc A1 (-87.5, 21) -> (-91.5, 17) centre (-87.5, 17) ccw
  line L3 (-5.5, 0) -> (5.5, 0)
  arc A2 (-9.5, 4) -> (-5.5, 0) centre (-5.5, 4) ccw
  line L4 (9.5, 4) -> (9.5, 36)
  line L5 (5.5, 40) -> (-106.5, 40)
  arc A3 (5.5, 0) -> (9.5, 4) centre (5.5, 4) ccw
  arc A4 (-95.5, 0) -> (-91.5, 4) centre (-95.5, 4) ccw
  arc A5 (-106.5, 40) -> (-110.5, 36) centre (-106.5, 36) ccw
  arc A6 (-110.5, 4) -> (-106.5, 0) centre (-106.5, 4) ccw
  arc A7 (-9.5, 17) -> (-13.5, 21) centre (-13.5, 17) ccw
  line L6 (-91.5, 4) -> (-91.5, 17)
  line L7 (-110.5, 36) -> (-110.5, 4)
  line L8 (-106.5, 32) -> (-106.5, 8)
  line L9 (-102.5, 4) -> (-99.5, 4)
  line L10 (-95.5, 8) -> (-95.5, 17)
  arc A8 (-87.5, 25) -> (-95.5, 17) centre (-87.5, 17) ccw
  line L11 (-87.5, 25) -> (-13.5, 25)
  arc A9 (-5.5, 17) -> (-13.5, 25) centre (-13.5, 17) ccw
  line L12 (-5.5, 17) -> (-5.5, 8)
  line L13 (-1.5, 4) -> (1.5, 4)
  line L14 (5.5, 8) -> (5.5, 32)
  line L15 (1.5, 36) -> (-102.5, 36)
  arc A10 (-102.5, 36) -> (-106.5, 32) centre (-102.5, 32) ccw
  arc A11 (-106.5, 8) -> (-102.5, 4) centre (-102.5, 8) ccw
  arc A12 (5.5, 32) -> (1.5, 36) centre (1.5, 32) ccw
  arc A13 (-5.5, 8) -> (-1.5, 4) centre (-1.5, 8) ccw
  arc A14 (1.5, 4) -> (5.5, 8) centre (1.5, 8) ccw
  arc A15 (-99.5, 4) -> (-95.5, 8) centre (-99.5, 8) ccw
  point P0 (-110.5, 40)
  point P1 (-9.5, 21)
  point P2 (-91.5, 21)
  point P3 (-91.5, 0)
  point P4 (9.5, 0)
  point P5 (9.5, 40)
  dimension "d336" = 120
  dimension "d337" = 40
  dimension "d338" = 82
  dimension "d339" = 21
  dimension "d340" = 4
  dimension "d341" = 4
  dimension "d342" = 4
  dimension "d343" = 4
  dimension "d344" = 4
  dimension "d345" = 4
  dimension "d346" = 4
  dimension "d347" = 4
  dimension "d368" = 4
  dimension "d369" = 4
  dimension "d370" = 4
  dimension "d371" = 4
  dimension "d372" = 4
  dimension "d373" = 4
  dimension "d374" = 5.5
  constraint horizontal L2
  constraint perpendicular L3 L4
  constraint parallel L2 L5
  constraint parallel L4 L7
  constraint horizontal L0
  constraint vertical L1
  constraint vertical L6
  constraint collinear L2 L3
  constraint coincident P3 L6
  constraint coincident P3 L2
  constraint tangent A4 L6
  constraint tangent L2 A4
  constraint tangent A6 L7
  constraint tangent L2 A6
  constraint coincident P0 L5
  constraint coincident P0 L7
  constraint tangent L5 A5
  constraint tangent A5 L7
  constraint coincident P2 L0
  constraint coincident P2 L6
  constraint tangent L0 A1
  constraint tangent A1 L6
  constraint coincident P1 L0
  constraint coincident P1 L1
  constraint tangent L0 A7
  constraint tangent L1 A7
  constraint coincident P5 L4
  constraint coincident P5 L5
  constraint tangent A0 L4
  constraint tangent A0 L5
  constraint coincident origin L3
  constraint coincident P4 L4
  constraint coincident P4 L3
  constraint tangent L4 A3
  constraint tangent L3 A3
  constraint tangent L1 A2
  constraint tangent L3 A2
  constraint equal L2 L3
  constraint concentric A1 A8
  constraint concentric A7 A9
  constraint tangent A9 L12
  constraint tangent L11 A9
  constraint tangent A8 L11
  constraint tangent L10 A8
  constraint tangent L8 A10
  constraint tangent L15 A10
  constraint tangent L8 A11
  constraint tangent L9 A11
  constraint tangent L14 A12
  constraint tangent L15 A12
  constraint tangent L12 A13
  constraint tangent L13 A13
  constraint tangent L13 A14
  constraint tangent L14 A14
  constraint tangent L9 A15
  constraint tangent L10 A15
  constraint collinear origin P3 P4
  measures "d336" distance of P0 P5
  measures "d337" distance of P4 P5
  measures "d338" distance of P1 P2
  measures "d339" distance of P2 P3
  measures "d340" radius of A4
  measures "d341" radius of A6
  measures "d342" radius of A5
  measures "d343" radius of A1
  measures "d344" radius of A7
  measures "d345" radius of A0
  measures "d346" radius of A3
  measures "d347" radius of A2
  measures "d368" radius of A10
  measures "d369" radius of A11
  measures "d370" radius of A12
  measures "d371" radius of A13
  measures "d372" radius of A14
  measures "d373" radius of A15
  measures "d374" horizontal distance of origin A3.centre